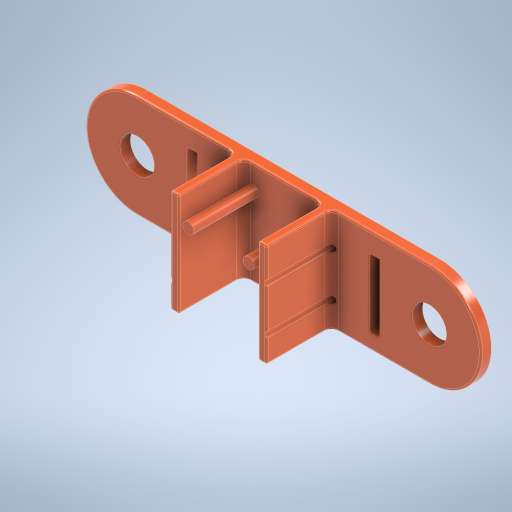
# Autodesk Inventor part: bişeyleramabendeisimveremedim
Saved by Autodesk Inventor 2023.2 (Build 272271000, 271)
## iProperties
Created: 2022-11-26
Part Number: bişeyleramabendeisimveremedim
Material: Generic
Document SubType Name: Modeling
Designer: omrfrkmll
Density: 1 g/cm^3
Appearance: Smooth - Light Orange
Author: omrfrkmll
Autodesk Inventor part; units mm, degrees
note: some values were not read from the file. Chosen so that the rebuilt part matches the saved one: direction of "Hole2".
ref_plane "YZ Plane" through (0, 0, 0) normal (1, 0, 0) x (0, 1, 0)
sketch "Sketch1" plane through (0, 0, 0) normal (0, 0, 1) x (1, 0, 0)
  line L0 (0, 7.8571) -> (0, -6.2528)
  line L1 (-7.0343, 0) -> (9.4203, 0)
  line L2 (-42.5, 15) -> (42.5, 15)
  line L3 (57.5, 0) -> (57.5, 0)
  line L4 (42.5, -15) -> (-42.5, -15)
  line L5 (-57.5, 0) -> (-57.5, 0)
  line L6 (25, 9.2468) -> (25, -10.7532)
  line L7 (-25, 9.4992) -> (-25, -10.5008)
  line L8 (-28, 9.4992) -> (-28, -10.5008)
  line L9 (28, 9.2468) -> (28, -10.7532)
  line L10 (-28, 9.4992) -> (-25, 9.4992)
  line L11 (-28, -10.5008) -> (-25, -10.5008)
  line L12 (25, -10.7532) -> (28, -10.7532)
  line L13 (25, 9.2468) -> (28, 9.2468)
  arc A0 (57.5, 0) -> (42.5, 15) centre (42.5, 0) ccw
  arc A1 (42.5, -15) -> (57.5, 0) centre (42.5, 0) ccw
  arc A2 (-57.5, 0) -> (-42.5, -15) centre (-42.5, 0) ccw
  arc A3 (-42.5, 15) -> (-57.5, 0) centre (-42.5, 0) ccw
  point P0 (0, 0)
  point P1 (-57.5, 15)
  point P2 (57.5, -15)
  point P3 (57.5, 15)
  point P4 (-57.5, -15)
  point P5 (-57.5, 0)
  dimension "d0" = 115
  dimension "d1" = 30
  dimension "d2" = 50
  dimension "d3" = 3
  dimension "d4" = 3
  dimension "d5" = 20
  dimension "d8" = 15
  constraints: 28 end point, 8 point on circle, 8 point on line, 8 tangent, 7 parallel, 4 centre point, 4 horizontal, 4 vertical, 3 equal radius, 2 perpendicular, 3 other
  measures "d0" distance between parallel lines of L3 L5
  measures "d1" distance between parallel lines of L4 L2
  measures "d2" distance between parallel lines of L6 L7
  measures "d3" distance between parallel lines of L7 L8
  measures "d4" distance between parallel lines of L6 L9
  measures "d5" distance between parallel lines of L11 L10
  measures "d8" radius of A0
extrude "Extrusion1" add sketch "Sketch1" along normal blind 3
sketch "Sketch12" plane through (0, 0, 3) normal (0, 0, 1) x (1, 0, 0)
  circle A0 centre (0, -12) radius 3.5
  circle A1 centre (-8.75, 8.0499) radius 1.6
  circle A2 centre (8.75, 8.0499) radius 1.6
  line L0 (0, 0) -> (-2.8557, 0)
  line L1 (0, 0) -> (0, -17)
  point P0 (0, -8.5)
  dimension "d87" = 7
  dimension "d88" = 21.876
  dimension "d89" = 21.876
  dimension "d90" = 3.2
  dimension "d91" = 12
  dimension "d98" = 17.5
  constraints: 4 end point, 2 centre point, 2 point on line, 1 equal radius, 1 midpoint, 1 vertical alignment, 3 other
  measures "d88" distance of A1.centre point (0, -12)
  measures "d89" distance of A2.centre point (0, -12)
  measures "d90" diameter of A2
  measures "d91" distance of point (0, 0) point (0, -12)
  measures "d98" distance of A2.centre A1.centre
extrude "Extrusion9" add sketch "Sketch12" along normal blind 18.85 contours A1 | A2
sketch "Sketch2" plane through (0, 0, 3) normal (0, 0, 1) x (1, 0, 0)
  arc A0 (42.5, -15) -> (42.5, 15) centre (42.5, 0) ccw projected
  arc A1 (-42.5, 15) -> (-42.5, -15) centre (-42.5, 0) ccw projected
  point P0 (0, 0)
  constraints: 2 coincident
hole "Hole1" at (42.5, 0, 3) at (-42.5, 0, 3) direction (0, 0, -1) diameter 10 end through all
ref_plane "Work Plane1" through (22, -10.7532, 0) normal (1, 0, 0) x (0, 0, -1)
sketch "Sketch7" plane through (0, 0, 0) normal (0, 0, -1) x (-1, 0, 0)
  line L0 (-33.9116, -11.0969) -> (-50.3989, -11.0969) construction
  line L1 (-50.3989, -11.0969) -> (-50.3989, -6.9201) construction
  line L2 (-50.3989, -6.9201) -> (-33.9116, -6.9201) construction
  line L3 (-33.9116, -6.9201) -> (-33.9116, -11.0969) construction
  spline S0 degree 2 poles (-35.2849, -6.9201) (-35.0157, -6.9201) (-34.6155, -7.0609) (-34.4747, -7.2017) knots 0 0 0 1 2 2 2
  spline S1 degree 2 poles (-34.4747, -7.2017) (-34.3142, -7.3598) (-34.1833, -7.8044) (-34.1833, -8.1304) knots 0 0 0 1 2 2 2
  line L4 (-34.1833, -8.1304) -> (-34.1833, -10.0323)
  line L5 (-34.1833, -10.0323) -> (-34.5884, -10.0323)
  line L6 (-34.5884, -10.0323) -> (-34.5884, -8.1304)
  spline S2 degree 2 poles (-34.5884, -8.1304) (-34.5884, -7.918) (-34.6427, -7.6315) (-34.7193, -7.5154) knots 0 0 0 1 2 2 2
  spline S3 degree 2 poles (-34.7193, -7.5154) (-34.8008, -7.3919) (-35.0824, -7.2659) (-35.2849, -7.2659) knots 0 0 0 1 2 2 2
  spline S4 degree 2 poles (-35.2849, -7.2659) (-35.4751, -7.2659) (-35.7715, -7.3919) (-35.853, -7.5154) knots 0 0 0 1 2 2 2
  spline S5 degree 2 poles (-35.853, -7.5154) (-35.9296, -7.6315) (-35.9839, -7.9155) (-35.9839, -8.1206) knots 0 0 0 1 2 2 2
  line L7 (-35.9839, -8.1206) -> (-35.9839, -10.0323)
  line L8 (-35.9839, -10.0323) -> (-36.389, -10.0323)
  line L9 (-36.389, -10.0323) -> (-36.389, -8.1304)
  spline S6 degree 2 poles (-36.389, -8.1304) (-36.389, -7.8118) (-36.2606, -7.3573) (-36.0975, -7.2017) knots 0 0 0 1 2 2 2
  spline S7 degree 2 poles (-36.0975, -7.2017) (-35.9518, -7.0584) (-35.5665, -6.9201) (-35.2849, -6.9201) knots 0 0 0 1 2 2 2
  line L10 (-35.1219, -10.4177) -> (-34.7094, -10.4177)
  line L11 (-34.7094, -10.4177) -> (-34.7094, -10.8178)
  line L12 (-34.7094, -10.8178) -> (-35.1219, -10.8178)
  line L13 (-35.1219, -10.8178) -> (-35.1219, -10.4177)
  line L14 (-35.9666, -10.4177) -> (-35.5541, -10.4177)
  line L15 (-35.5541, -10.4177) -> (-35.5541, -10.8178)
  line L16 (-35.5541, -10.8178) -> (-35.9666, -10.8178)
  line L17 (-35.9666, -10.8178) -> (-35.9666, -10.4177)
  spline S8 degree 2 poles (-37.8191, -6.93) (-37.4882, -6.93) (-37.0238, -7.0683) (-36.8188, -7.1671) knots 0 0 0 1 2 2 2
  line L18 (-36.8188, -7.1671) -> (-36.8188, -7.676)
  line L19 (-36.8188, -7.676) -> (-36.8484, -7.676)
  spline S9 degree 2 poles (-36.8484, -7.676) (-37.0485, -7.4882) (-37.5549, -7.2808) (-37.7895, -7.2808) knots 0 0 0 1 2 2 2
  spline S10 degree 2 poles (-37.7895, -7.2808) (-38.1254, -7.2808) (-38.4688, -7.5599) (-38.4688, -7.7896) knots 0 0 0 1 2 2 2
  spline S11 degree 2 poles (-38.4688, -7.7896) (-38.4688, -7.9724) (-38.2885, -8.1996) (-38.0933, -8.2564) knots 0 0 0 1 2 2 2
  spline S12 degree 2 poles (-38.0933, -8.2564) (-37.9525, -8.2959) (-37.7179, -8.3503) (-37.5425, -8.3947) knots 0 0 0 1 2 2 2
  spline S13 degree 2 poles (-37.5425, -8.3947) (-37.3844, -8.4367) (-37.135, -8.5627) (-37.0386, -8.664) knots 0 0 0 1 2 2 2
  spline S14 degree 2 poles (-37.0386, -8.664) (-36.9448, -8.7652) (-36.841, -9.0369) (-36.841, -9.2148) knots 0 0 0 1 2 2 2
  spline S15 degree 2 poles (-36.841, -9.2148) (-36.841, -9.5853) (-37.419, -10.0867) (-37.8661, -10.0867) knots 0 0 0 1 2 2 2
  spline S16 degree 2 poles (-37.8661, -10.0867) (-38.123, -10.0867) (-38.5774, -9.9854) (-38.7726, -9.8891) knots 0 0 0 1 2 2 2
  line L20 (-38.7726, -9.8891) -> (-38.7726, -9.405)
  line L21 (-38.7726, -9.405) -> (-38.7429, -9.405)
  spline S17 degree 2 poles (-38.7429, -9.405) (-38.5972, -9.5383) (-38.1427, -9.7359) (-37.8932, -9.7359) knots 0 0 0 1 2 2 2
  spline S18 degree 2 poles (-37.8932, -9.7359) (-37.6117, -9.7359) (-37.2634, -9.4717) (-37.2634, -9.2568) knots 0 0 0 1 2 2 2
  spline S19 degree 2 poles (-37.2634, -9.2568) (-37.2634, -9.0641) (-37.4684, -8.8344) (-37.6611, -8.7825) knots 0 0 0 1 2 2 2
  spline S20 degree 2 poles (-37.6611, -8.7825) (-37.7895, -8.7479) (-38.1625, -8.659) (-38.286, -8.622) knots 0 0 0 1 2 2 2
  spline S21 degree 2 poles (-38.286, -8.622) (-38.5997, -8.5256) (-38.8911, -8.1378) (-38.8911, -7.8538) knots 0 0 0 1 2 2 2
  spline S22 degree 2 poles (-38.8911, -7.8538) (-38.8911, -7.6735) (-38.7454, -7.3277) (-38.6145, -7.2066) knots 0 0 0 1 2 2 2
  spline S23 degree 2 poles (-38.6145, -7.2066) (-38.4688, -7.0733) (-38.0983, -6.93) (-37.8191, -6.93) knots 0 0 0 1 2 2 2
  line L22 (-40.015, -6.9843) -> (-40.015, -9.6717)
  line L23 (-40.015, -9.6717) -> (-38.9924, -9.6717)
  line L24 (-38.9924, -9.6717) -> (-38.9924, -10.0323)
  line L25 (-38.9924, -10.0323) -> (-41.4427, -10.0323)
  line L26 (-41.4427, -10.0323) -> (-41.4427, -9.6717)
  line L27 (-41.4427, -9.6717) -> (-40.4201, -9.6717)
  line L28 (-40.4201, -9.6717) -> (-40.4201, -6.9843)
  line L29 (-40.4201, -6.9843) -> (-40.015, -6.9843)
  spline S24 degree 2 poles (-43.9102, -6.93) (-43.5792, -6.93) (-43.1149, -7.0683) (-42.9099, -7.1671) knots 0 0 0 1 2 2 2
  line L30 (-42.9099, -7.1671) -> (-42.9099, -7.676)
  line L31 (-42.9099, -7.676) -> (-42.9395, -7.676)
  spline S25 degree 2 poles (-42.9395, -7.676) (-43.1396, -7.4882) (-43.6459, -7.2808) (-43.8806, -7.2808) knots 0 0 0 1 2 2 2
  spline S26 degree 2 poles (-43.8806, -7.2808) (-44.2165, -7.2808) (-44.5598, -7.5599) (-44.5598, -7.7896) knots 0 0 0 1 2 2 2
  spline S27 degree 2 poles (-44.5598, -7.7896) (-44.5598, -7.9724) (-44.3795, -8.1996) (-44.1844, -8.2564) knots 0 0 0 1 2 2 2
  spline S28 degree 2 poles (-44.1844, -8.2564) (-44.0436, -8.2959) (-43.8089, -8.3503) (-43.6336, -8.3947) knots 0 0 0 1 2 2 2
  spline S29 degree 2 poles (-43.6336, -8.3947) (-43.4755, -8.4367) (-43.226, -8.5627) (-43.1297, -8.664) knots 0 0 0 1 2 2 2
  spline S30 degree 2 poles (-43.1297, -8.664) (-43.0358, -8.7652) (-42.9321, -9.0369) (-42.9321, -9.2148) knots 0 0 0 1 2 2 2
  spline S31 degree 2 poles (-42.9321, -9.2148) (-42.9321, -9.5853) (-43.5101, -10.0867) (-43.9571, -10.0867) knots 0 0 0 1 2 2 2
  spline S32 degree 2 poles (-43.9571, -10.0867) (-44.214, -10.0867) (-44.6685, -9.9854) (-44.8636, -9.8891) knots 0 0 0 1 2 2 2
  line L32 (-44.8636, -9.8891) -> (-44.8636, -9.405)
  line L33 (-44.8636, -9.405) -> (-44.834, -9.405)
  spline S33 degree 2 poles (-44.834, -9.405) (-44.6883, -9.5383) (-44.2338, -9.7359) (-43.9843, -9.7359) knots 0 0 0 1 2 2 2
  spline S34 degree 2 poles (-43.9843, -9.7359) (-43.7027, -9.7359) (-43.3545, -9.4717) (-43.3545, -9.2568) knots 0 0 0 1 2 2 2
  spline S35 degree 2 poles (-43.3545, -9.2568) (-43.3545, -9.0641) (-43.5595, -8.8344) (-43.7521, -8.7825) knots 0 0 0 1 2 2 2
  spline S36 degree 2 poles (-43.7521, -8.7825) (-43.8806, -8.7479) (-44.2535, -8.659) (-44.377, -8.622) knots 0 0 0 1 2 2 2
  spline S37 degree 2 poles (-44.377, -8.622) (-44.6907, -8.5256) (-44.9822, -8.1378) (-44.9822, -7.8538) knots 0 0 0 1 2 2 2
  spline S38 degree 2 poles (-44.9822, -7.8538) (-44.9822, -7.6735) (-44.8365, -7.3277) (-44.7056, -7.2066) knots 0 0 0 1 2 2 2
  spline S39 degree 2 poles (-44.7056, -7.2066) (-44.5598, -7.0733) (-44.1893, -6.93) (-43.9102, -6.93) knots 0 0 0 1 2 2 2
  line L34 (-45.0662, -6.9843) -> (-46.0937, -10.0323)
  line L35 (-46.0937, -10.0323) -> (-46.5926, -10.0323)
  line L36 (-46.5926, -10.0323) -> (-47.6202, -6.9843)
  line L37 (-47.6202, -6.9843) -> (-47.1929, -6.9843)
  line L38 (-47.1929, -6.9843) -> (-46.9162, -7.8365)
  line L39 (-46.9162, -7.8365) -> (-45.7528, -7.8365)
  line L40 (-45.7528, -7.8365) -> (-45.4762, -6.9843)
  line L41 (-45.4762, -6.9843) -> (-45.0662, -6.9843)
  line L42 (-46.8051, -8.1823) -> (-46.3333, -9.6174)
  line L43 (-46.3333, -9.6174) -> (-45.864, -8.1823)
  line L44 (-45.864, -8.1823) -> (-46.8051, -8.1823)
  spline S40 degree 2 poles (-49.1862, -6.9251) (-48.8626, -6.9251) (-48.3266, -7.1227) (-48.1339, -7.3227) knots 0 0 0 1 2 2 2
  spline S41 degree 2 poles (-48.1339, -7.3227) (-47.9413, -7.5253) (-47.7363, -8.123) (-47.7363, -8.5108) knots 0 0 0 1 2 2 2
  spline S42 degree 2 poles (-47.7363, -8.5108) (-47.7363, -8.8789) (-47.9437, -9.4618) (-48.1364, -9.6693) knots 0 0 0 1 2 2 2
  spline S43 degree 2 poles (-48.1364, -9.6693) (-48.3217, -9.8693) (-48.8651, -10.0867) (-49.1886, -10.0867) knots 0 0 0 1 2 2 2
  spline S44 degree 2 poles (-49.1886, -10.0867) (-49.3442, -10.0867) (-49.6258, -10.0422) (-49.7543, -10.0027) knots 0 0 0 1 2 2 2
  spline S45 degree 2 poles (-49.7543, -10.0027) (-49.858, -9.9731) (-50.1099, -9.8644) (-50.1865, -9.8249) knots 0 0 0 1 2 2 2
  line L45 (-50.1865, -9.8249) -> (-50.1865, -9.3358)
  line L46 (-50.1865, -9.3358) -> (-50.1519, -9.3358)
  spline S46 degree 2 poles (-50.1519, -9.3358) (-50.0754, -9.4025) (-49.9148, -9.5235) (-49.7666, -9.5927) knots 0 0 0 1 2 2 2
  spline S47 degree 2 poles (-49.7666, -9.5927) (-49.6431, -9.6544) (-49.3245, -9.7359) (-49.1417, -9.7359) knots 0 0 0 1 2 2 2
  spline S48 degree 2 poles (-49.1417, -9.7359) (-48.702, -9.7359) (-48.1586, -9.074) (-48.1586, -8.5232) knots 0 0 0 1 2 2 2
  spline S49 degree 2 poles (-48.1586, -8.5232) (-48.1586, -8.2169) (-48.3019, -7.7575) (-48.4377, -7.5994) knots 0 0 0 1 2 2 2
  spline S50 degree 2 poles (-48.4377, -7.5994) (-48.5687, -7.4413) (-48.9392, -7.2758) (-49.1713, -7.2758) knots 0 0 0 1 2 2 2
  spline S51 degree 2 poles (-49.1713, -7.2758) (-49.3418, -7.2758) (-49.6826, -7.3252) (-49.7987, -7.3746) knots 0 0 0 1 2 2 2
  line L47 (-49.7987, -7.3746) -> (-49.7987, -8.1625)
  line L48 (-49.7987, -8.1625) -> (-49.0923, -8.1625)
  line L49 (-49.0923, -8.1625) -> (-49.0923, -8.5182)
  line L50 (-49.0923, -8.5182) -> (-50.1989, -8.5182)
  line L51 (-50.1989, -8.5182) -> (-50.1989, -7.1869)
  spline S52 degree 2 poles (-50.1989, -7.1869) (-50.1223, -7.1523) (-49.8605, -7.0461) (-49.7493, -7.014) knots 0 0 0 1 2 2 2
  spline S53 degree 2 poles (-49.7493, -7.014) (-49.5987, -6.9695) (-49.3566, -6.9251) (-49.1862, -6.9251) knots 0 0 0 1 2 2 2
  spline S54 degree 2 poles (-49.7839, -11.0969) (-49.7839, -10.9216) (-49.6975, -10.6326) (-49.6184, -10.5338) knots 0 0 0 1 2 2 2
  spline S55 degree 2 poles (-49.6184, -10.5338) (-49.527, -10.4251) (-49.2924, -10.3164) (-49.1096, -10.3164) knots 0 0 0 1 2 2 2
  spline S56 degree 2 poles (-49.1096, -10.3164) (-48.9416, -10.3164) (-48.6922, -10.43) (-48.6057, -10.5338) knots 0 0 0 1 2 2 2
  spline S57 degree 2 poles (-48.6057, -10.5338) (-48.5217, -10.635) (-48.4353, -10.924) (-48.4353, -11.0969) knots 0 0 0 1 2 2 2
  line L52 (-48.4353, -11.0969) -> (-48.7663, -11.0969)
  spline S58 degree 2 poles (-48.7663, -11.0969) (-48.7663, -10.8203) (-48.9392, -10.5758) (-49.1096, -10.5758) knots 0 0 0 1 2 2 2
  spline S59 degree 2 poles (-49.1096, -10.5758) (-49.2726, -10.5758) (-49.4529, -10.8153) (-49.4529, -11.0969) knots 0 0 0 1 2 2 2
  line L53 (-49.4529, -11.0969) -> (-49.7839, -11.0969)
  point P0 (0, 0)
  constraints: 2 other
emboss "Emboss1" sketch "Sketch7" operation cut depth 1 direction (0, 0, 1)
ref_plane "Work Plane2" through (-31, -10.5008, 0) normal (1, 0, 0) x (0, 0, -1)
sketch "Sketch10" plane through (0, 0, 3) normal (0, 0, 1) x (1, 0, 0)
  line L0 (0, 0) -> (0, 20.7608)
  line L1 (0, 0) -> (9.282, 0)
  line L2 (-14, 15) -> (14, 15)
  line L3 (11.5, 15) -> (11.5, -15)
  line L4 (14, -15) -> (-14, -15)
  line L5 (-11.5, -15) -> (-11.5, 15)
  line L6 (42.5, 15) -> (-42.5, 15) projected
  line L7 (14, 15) -> (14, -15)
  line L8 (-14, -15) -> (-14, 15)
  line L9 (-42.5, -15) -> (42.5, -15) projected
  point P0 (0, 15)
  point P1 (0, -15)
  dimension "d83" = 23
  dimension "d84" = 2.5
  dimension "d100" = 2.5
  constraints: 16 end point, 7 point on line, 4 midpoint, 3 parallel, 2 horizontal, 1 perpendicular, 1 vertical, 1 other
  measures "d83" distance between parallel lines of L3 L5
  measures "d84" distance between parallel lines of L5 L8
  measures "d100" distance between parallel lines of L7 L3
extrude "Extrusion8" add sketch "Sketch10" along normal blind 18.85 contours L2 L5 L4 L8 | L2 L7 L4 L3
fillet "Fillet9" radius 2 4 edges at (-14, 0, 3) (14, 0, 3) (11.5, 0, 3) (-11.5, 0, 3)
extrude "Extrusion10" cut sketch "Sketch12" against normal up to surface (3 mm away) contours A0 L1 | L1 A0
fillet "Fillet10" radius 2 2 edges at (-1.8028, -15, 1.5) (1.8028, -15, 1.5)
fillet "Fillet11" radius 0.5 36 edges at (-14, 0, 21.85) (-11.5, 0, 21.85) (11.5, 0, 21.85) (14, 0, 21.85) (12.75, -15, 21.85) (12.75, 15, 21.85) (-12.75, 15, 21.85) (-12.75, -15, 21.85) (-14.5858, -15, 3.5858) (-29.25, -15, 3) (-57.5, 0, 3) (-29.25, 15, 3) (-14.5858, 15, 3.5858) (-14, 15, 13.425) (-14, -15, 13.425) (-10.9142, -15, 3.5858) (-7.4542, -15, 3) (7.4542, -15, 3) (-3.8709, -14.2792, 3) (3.8709, -14.2792, 3) (0, -8.5, 3) (10.9142, -15, 3.5858) (11.5, -15, 13.425) (-11.5, -15, 13.425) (14.5858, -15, 3.5858) (29.25, -15, 3) (57.5, 0, 3) (29.25, 15, 3) (14.5858, 15, 3.5858) (14, 15, 13.425) (14, -15, 13.425) (-10.9142, 15, 3.5858) (-11.5, 15, 13.425) (10.9142, 15, 3.5858) (11.5, 15, 13.425) (0, 15, 3)
sketch "Sketch13" plane through (0, 0, 0) normal (0, 0, -1) x (-1, 0, 0)
  circle A0 centre (-42.5, 0) radius 5 projected
  line L0 (-14.5003, -7.501) -> (-14.5003, 20.5498)
  line L1 (-42.5, 15) -> (42.5, 15) projected
  line L2 (0, 0) -> (0, -18.5385)
  line L3 (-5.4083, -15) -> (-42.5, -15) projected
  point P0 (-14.5003, 5.499)
  point P1 (14.5003, -7.501)
  point P2 (14.5003, 5.499)
  dimension "d103" = 13
  dimension "d111" = 20.499
  dimension "d112" = 28.987
  constraints: 4 end point, 2 symmetric about line, 2 vertical, 1 point on line
  measures "d103" distance of L0.start point (-14.5, 5.499)
  measures "d111" distance from line of L3 point (-14.5, 5.499)
  measures "d112" distance of A0.centre L0.start
hole "Hole2" at (14.5003, -7.501, 0) at (14.5003, 5.499, 0) at (-14.5003, -7.501, 0) at (-14.5003, 5.499, 0) direction (0, 0, 1) diameter 2.1 depth 21.85
body "Solid1"
